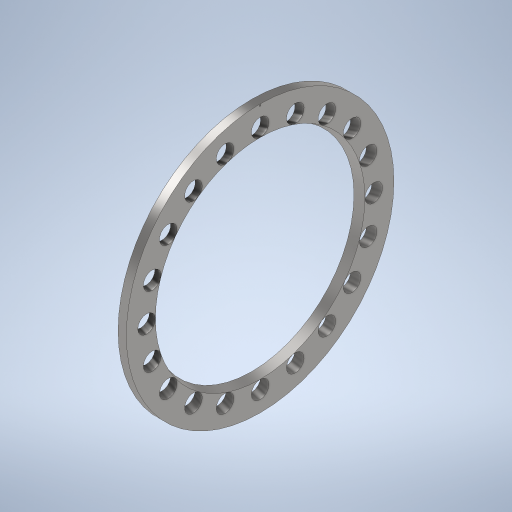
# Autodesk Inventor part: back bracket 2
Saved by Autodesk Inventor 2023 (Build 270158000, 158)
## iProperties
Created: 2022-07-22
Part Number: back bracket 2
Material: Stainless Steel
Document SubType Name: Modeling
Designer: station
Density: 8 g/cm^3
Appearance: Semi-Polished
Mass: 75.6084 g
Surface Area: 87.9822 cm^2
Volume: 9.45105 cm^3
Author: station
Autodesk Inventor part; units mm, degrees
ref_plane "YZ Plane" through (0, 0, 0) normal (1, 0, 0) x (0, 1, 0)
ref_plane "XZ Plane" through (0, 0, 0) normal (0, 1, 0) x (-1, 0, 0)
ref_plane "XY Plane" through (0, 0, 0) normal (0, 0, 1) x (1, 0, 0)
sketch "Sketch1" plane through (0, 0, 0) normal (0, 0, 1) x (1, 0, 0)
  arc A0 (180.1312, 23.4516) -> (181.5833, 23.6751) centre (180.1312, 28.2803) ccw
  arc A1 (180.1312, 23.4516) -> (181.5842, 23.6753) centre (180.1312, 28.2803) ccw
  arc A2 (180.1312, 21.4516) -> (182.1847, 21.7676) centre (180.1312, 28.2803) ccw
  arc A3 (167.724, 26.7761) -> (180.1312, 23.4516) centre (180.1312, 48.266) ccw
  arc A4 (166.724, 25.044) -> (180.1312, 21.4516) centre (180.1312, 48.266) ccw
  arc A5 (166.724, 49.052) -> (167.724, 48.052) centre (167.724, 49.052) ccw
  line L0 (234.2883, 48.052) -> (167.724, 48.052)
  line L1 (234.2883, 50.052) -> (169.724, 50.052)
  line L2 (182.1847, 21.7676) -> (237.115, 39.0871)
  line L3 (236.5136, 40.9945) -> (181.5833, 23.6751)
  line L4 (168.724, 21.0384) -> (168.724, 27.7779)
  line L5 (166.724, 21.0384) -> (166.724, -8.65)
  line L6 (236.5136, 40.9945) -> (237.115, 39.0871)
  line L7 (234.2883, 48.052) -> (238.3779, 48.052)
  line L8 (234.2883, 50.052) -> (238.3779, 50.052)
  line L9 (238.3779, 48.052) -> (238.3779, 50.052)
  line L10 (0, -0.4301) -> (319.1694, -0.4301)
  line L11 (0, 80.4749) -> (30.0219, 80.4749)
  line L12 (30.0219, 82.4749) -> (0, 82.4749)
  line L13 (0, 80.4749) -> (0, 82.4749)
  line L14 (0, 73.0749) -> (30.0219, 73.0749)
  line L15 (0, 71.0749) -> (30.0219, 71.0749)
  line L16 (124.3912, 47.7887) -> (167.724, 22.7705)
  line L17 (123.3912, 46.0566) -> (166.724, 21.0384)
  line L18 (166.724, 21.0384) -> (166.724, 27.1473)
  arc A6 (123.3912, 46.0566) -> (30.0219, 71.0749) centre (30.0219, -115.6637) ccw
  arc A7 (124.3912, 47.7887) -> (30.0219, 73.0749) centre (30.0219, -115.6637) ccw
  line L19 (30.0219, 80.4749) -> (165.724, 80.4749)
  line L20 (167.724, 82.4749) -> (30.0219, 82.4749)
  line L21 (166.724, 49.052) -> (166.724, 79.4749)
  line L22 (168.724, 51.052) -> (168.724, 81.4749)
  arc A8 (168.724, 51.052) -> (169.724, 50.052) centre (169.724, 51.052) ccw
  arc A9 (166.724, 79.4749) -> (165.724, 80.4749) centre (165.724, 79.4749) ccw
  arc A10 (168.724, 81.4749) -> (167.724, 82.4749) centre (167.724, 81.4749) ccw
  line L23 (236.5136, 40.9945) -> (236.5136, 48.052)
  line L24 (236.5136, 48.052) -> (233.5136, 48.052)
  line L25 (233.5136, 48.052) -> (233.5136, 40.0486)
  line L26 (233.5136, 48.052) -> (225.5136, 48.052)
  line L27 (225.5136, 48.052) -> (225.5136, 37.5262)
  line L28 (225.5136, 48.052) -> (222.5136, 48.052)
  line L29 (222.5136, 48.052) -> (222.5136, 36.5803)
  line L30 (234.2883, 48.052) -> (225.5136, 45.6835)
  line L31 (222.5136, 44.7377) -> (144.4694, 20.1304)
  dimension "d18" = 30.0219
  dimension "d19" = 186.7386
  dimension "d20" = 0
  dimension "d21" = 0
  dimension "d22" = 71.505
  dimension "d23" = 2
  dimension "d24" = 2
  dimension "d25" = 2
  dimension "d26" = 2
  dimension "d27" = 2
  dimension "d28" = 17.5
  dimension "d29" = 54.9303
  dimension "d30" = 2
  dimension "d31" = 7.4
  dimension "d32" = 7.4
  dimension "d34" = 2
  dimension "d35" = 2
  dimension "d36" = 1
  dimension "d37" = 1
  dimension "d38" = 1
  dimension "d39" = 1
  dimension "d40" = 3
  dimension "d41" = 8
  dimension "d42" = 3
  constraints: 64 end point, 22 point on circle, 11 centre point, 11 point on line, 9 tangent, 5 perpendicular, 4 horizontal, 4 parallel, 4 vertical, 2 other
  measures "d18" distance of L15.start L15.end
  measures "d19" radius of A6
  measures "d20" distance of A6.end L15.end
  measures "d21" distance of L17.start A6.start
  measures "d22" distance between parallel lines of L10 L15
  measures "d23" distance between parallel lines of L15 L14
  measures "d24" radial gap between concentric circles of A6 A7
  measures "d25" distance between parallel lines of L17 L16
  measures "d26" radial gap between concentric circles of A4 A3
  measures "d27" radial gap between concentric circles of A2 A1
  measures "d28" angle of L10 L2
  measures "d29" horizontal distance of L2.start L2.end
  measures "d30" distance between parallel lines of L2 L3
  measures "d31" distance between parallel lines of L14 L11
  measures "d32" distance of L0.start L3.start
  measures "d34" distance between parallel lines of L19 L20
  measures "d35" distance between parallel lines of L0 L1
  measures "d36" radius of A9
  measures "d37" radius of A10
  measures "d38" radius of A8
  measures "d39" radius of A5
  measures "d40" distance of L23.end L25.start
  measures "d41" distance of L25.start L26.end
  measures "d42" distance of L26.end L28.end
revolve "Revolution1" add sketch "Sketch1" angle 360 about axis through (0, -0.4301, 0) along (1, 0, 0) contours L29 L0 L27 L3
sketch "Sketch4" plane through (225.5136, -0.4301, 0) normal (1, 0, 0) x (0, 0, -1)
  circle A0 centre (0, 0) radius 37.9564 projected
  line L0 (0, 37.9564) -> (0, 41.1564)
  circle A1 centre (0, 41.1564) radius 3.2
  point P0 (0, 0.4301)
  dimension "d47" = 3.2
  dimension "d48" = 6.4
  constraints: 2 end point, 1 centre point, 1 coincident, 1 vertical, 1 vertical alignment, 1 other
  measures "d47" distance of L0.start L0.end
  measures "d48" diameter of A1
sketch "Sketch5" plane through (222.5136, -0.4301, 0) normal (-1, 0, 0) x (0, 0, 1)
  circle A0 centre (0, 0) radius 37.0105 projected
  line L0 (0, 37.0105) -> (0, 40.2105)
  circle A1 centre (0, 40.2105) radius 3.2
  point P0 (0, 0.4301)
  dimension "d49" = 3.2
  dimension "d50" = 6.4
  constraints: 2 end point, 1 centre point, 1 coincident, 1 vertical, 1 vertical alignment, 1 other
  measures "d49" distance of L0.start L0.end
  measures "d50" diameter of A1
sketch "Sketch6" plane through (0, 0, 0) normal (0, 0, 1) x (1, 0, 0)
  line L0 (225.5136, -48.9123) -> (225.5136, 48.052) projected
  line L1 (225.5136, 42.2627) -> (222.5136, 41.3779)
  line L2 (222.5136, -48.9123) -> (222.5136, 48.052) projected
  point P0 (0, 0)
  constraints: 2 end point, 2 point on line
sweep "Sweep1" cut profiles "Sketch4" path "Sketch6" path curves L1 contours A1
pattern_circular "Circular Pattern1" count 20 over 360 about axis through (224.0136, -0.4301, 0) along (1, 0, 0) of "Sweep1"
sketch "Sketch7" plane through (225.5136, -0.4301, 0) normal (1, 0, 0) x (0, 0, -1)
  circle A0 centre (0, 0) radius 48.4822 projected
  line L0 (0, 48.4822) -> (0, 47.9822)
  line L1 (0.25, 47.7322) -> (-0.25, 47.7322)
  line L2 (-0.25, 47.7322) -> (-0.25, 48.2322)
  line L3 (-0.25, 48.2322) -> (0.25, 48.2322)
  line L4 (0.25, 48.2322) -> (0.25, 47.7322)
  line L5 (0.25, 47.7322) -> (-0.25, 48.2322) construction
  line L6 (-0.25, 47.7322) -> (0.25, 48.2322) construction
  point P0 (0, 0.4301)
  dimension "d56" = 0.5
  dimension "d60" = 0.5
  dimension "d61" = 0.5
  constraints: 14 end point, 2 midpoint, 2 parallel, 1 horizontal, 1 perpendicular, 1 vertical, 1 vertical alignment, 1 other
  measures "d56" distance of L0.start L0.end
  measures "d60" distance of L2.end L3.end
  measures "d61" distance of L1.end L2.end
extrude "Extrusion1" cut sketch "Sketch7" against normal blind 10 contours L1 L2 L3 L4
body "Solid1"
